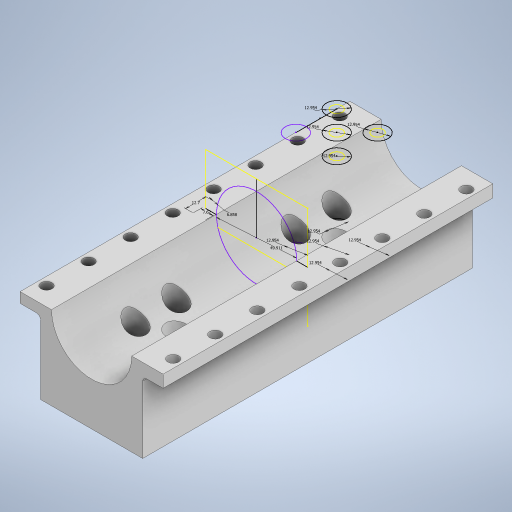
# Autodesk Inventor part: CameraHolder_LengthofTranslationStage
Saved by Autodesk Inventor 2024.2 (Build 282272000, 272)
## iProperties
Created: 2023-12-14
Part Number: CameraHolder_LengthofTranslationStage
Material: Generic
Document SubType Name: Modeling
Designer: S227943
Density: 1 g/cm^3
Appearance: Default
Author: S227943
Autodesk Inventor part; units mm, degrees
ref_plane "YZ Plane" through (0, 0, 0) normal (1, 0, 0) x (0, 1, 0)
ref_plane "XZ Plane" through (0, 0, 0) normal (0, 1, 0) x (-1, 0, 0)
ref_plane "XY Plane" through (0, 0, 0) normal (0, 0, 1) x (1, 0, 0)
sketch "Sketch1" plane through (0, 0, 0) normal (0, 1, 0) x (-1, 0, 0)
  line L0 (0, 0) -> (0, -102.499)
  line L1 (0, -102.499) -> (63.5, -102.499)
  line L2 (63.5, -102.499) -> (63.5, 0)
  line L3 (63.5, 0) -> (0, 0)
  dimension "d0" = 102.499
  dimension "d1" = 63.5
  constraints: 8 end point, 3 perpendicular, 1 vertical
  measures "d0" distance of L0.start L0.end
  measures "d1" distance of L0.end L1.end
extrude "Extrusion1" add sketch "Sketch1" along normal blind 63.5
sketch "Sketch2" plane through (-63.5, 0, 0) normal (0, 0, 1) x (1, 0, 0)
  line L0 (63.5, 63.5) -> (0, 63.5) projected
  line L1 (31.75, 63.5) -> (31.75, 31.75)
  circle A0 centre (31.75, 31.75) radius 24.9555
  line L2 (0, 0) -> (0, 63.5) projected
  line L3 (0, 31.75) -> (6.7945, 31.75)
  line L4 (63.5, 0) -> (63.5, 63.5) projected
  line L5 (63.5, 31.75) -> (56.7055, 31.75)
  dimension "d4" = 49.911
  constraints: 6 end point, 3 midpoint, 2 point on circle, 1 centre point, 1 coincident, 1 perpendicular, 1 point on line, 1 vertical
  measures "d4" diameter of A0
extrude "Extrusion2" cut sketch "Sketch2" against normal blind 139.7 contours A0
sketch "Sketch3" plane through (0, 0, 0) normal (1, 0, 0) x (0, 0, -1)
  line L0 (0, 0) -> (0, 63.5) projected
  line L1 (0, 31.75) -> (102.499, 31.75)
  line L2 (102.499, 0) -> (102.499, 63.5) projected
  constraints: 2 end point, 2 midpoint
split_face "Split1"
extrude "Extrusion3" cut sketch "Sketch2" against normal blind 139.7 contours L4 L5 A0 L1 L0 | L1 A0 L3 L2 L0
sketch "Sketch5" plane through (0, 0, 0) normal (0, -1, 0) x (1, 0, 0)
  line L0 (0, 0) -> (-31.75, 0)
  line L1 (-56.7055, 0) -> (-6.7945, 0) projected
  line L2 (-31.75, 0) -> (-31.75, -49.794)
  line L3 (0, 0) -> (0, -102.499) projected
  line L4 (-31.75, -49.794) -> (-19.05, -49.794)
  line L5 (-19.05, -49.794) -> (-19.05, -62.494)
  line L6 (-19.05, -62.494) -> (-44.45, -62.494)
  line L7 (-44.45, -62.494) -> (-44.45, -37.094)
  line L8 (-44.45, -37.094) -> (-19.05, -37.094)
  circle A0 centre (-19.05, -62.494) radius 3.429
  circle A1 centre (-44.45, -62.494) radius 3.429
  circle A2 centre (-19.05, -37.094) radius 3.429
  circle A3 centre (-44.45, -37.094) radius 3.429
  circle A4 centre (-31.75, -49.794) radius 3.429
  line L9 (-19.05, -62.494) -> (-19.05, -102.499)
  line L10 (0, -102.499) -> (-63.5, -102.499) projected
  dimension "d9" = 12.7
  dimension "d10" = 12.7
  dimension "d11" = 25.4
  dimension "d12" = 25.4
  dimension "d13" = 6.858
  dimension "d14" = 6.858
  dimension "d15" = 6.858
  dimension "d16" = 6.858
  dimension "d17" = 6.858
  dimension "d74" = 40.005
  constraints: 16 end point, 5 centre point, 5 coincident, 4 perpendicular, 2 point on line, 1 midpoint, 1 parallel, 1 vertical
  measures "d9" distance of L2.end L4.end
  measures "d10" distance of L4.end L5.end
  measures "d11" distance of L5.end L6.end
  measures "d12" distance of L6.end L7.end
  measures "d13" diameter of A0
  measures "d14" diameter of A1
  measures "d15" diameter of A2
  measures "d16" diameter of A3
  measures "d17" diameter of A4
  measures "d74" distance of L9.start L9.end
extrude "Extrusion4" cut sketch "Sketch5" against normal blind 139.7 contours L9 L5 A0 | A0 L6 L9 | A4 L4 L2 | L2 L4 A4 | A3 L7 L8 | L8 L7 A3 | A0 L5 L6 | A1 L7 L6 | L6 L7 A1 | A2
sketch "Sketch6" plane through (0, 0, 0) normal (0, -1, 0) x (1, 0, 0)
  circle A0 centre (-19.05, -37.094) radius 3.429 projected
  circle A1 centre (-44.45, -37.094) radius 3.429 projected
  line L0 (-19.05, -37.094) -> (-44.45, -37.094)
  circle A2 centre (-44.45, -62.494) radius 3.429 projected
  line L1 (-44.45, -37.094) -> (-44.45, -62.494)
  line L2 (-44.45, -62.494) -> (-19.05, -62.494)
  line L3 (-19.05, -62.494) -> (-31.75, -49.794)
  circle A3 centre (-19.05, -37.094) radius 6.477
  circle A4 centre (-31.75, -49.794) radius 6.477
  circle A5 centre (-44.45, -62.494) radius 6.477
  circle A6 centre (-19.05, -62.494) radius 6.477
  circle A7 centre (-44.45, -37.094) radius 6.477
  point P0 (0, 0)
  dimension "d20" = 12.954
  dimension "d21" = 12.954
  dimension "d22" = 12.954
  dimension "d23" = 12.954
  dimension "d24" = 12.954
  constraints: 8 end point, 5 centre point, 4 coincident, 2 perpendicular, 1 horizontal, 1 point on line
  measures "d20" diameter of A3
  measures "d21" diameter of A4
  measures "d22" diameter of A5
  measures "d23" diameter of A6
  measures "d24" diameter of A7
sketch "Sketch7" plane through (0, 63.5, 0) normal (0, 1, 0) x (1, 0, 0)
  circle A0 centre (-19.05, 37.094) radius 3.429 projected
  circle A1 centre (-19.05, 37.094) radius 6.477
  circle A2 centre (-31.75, 49.794) radius 3.429 projected
  circle A3 centre (-31.75, 49.794) radius 6.477
  circle A4 centre (-44.45, 62.494) radius 3.429 projected
  circle A5 centre (-44.45, 62.494) radius 6.477
  circle A6 centre (-19.05, 62.494) radius 3.429 projected
  circle A7 centre (-19.05, 62.494) radius 6.477
  line L0 (-44.45, 62.494) -> (-44.45, 52.2986)
  line L1 (-44.45, 62.494) -> (-44.45, 37.094)
  circle A8 centre (-44.45, 37.094) radius 6.477
  point P0 (0, 0)
  dimension "d25" = 12.954
  dimension "d26" = 12.954
  dimension "d28" = 12.954
  dimension "d29" = 12.954
  constraints: 5 centre point, 5 coincident, 4 end point, 2 vertical
  measures "d25" diameter of A1
  measures "d26" diameter of A3
  measures "d28" diameter of A5
  measures "d29" diameter of A7
extrude "Extrusion5" cut sketch "Sketch7" against normal blind 62.23 contours A0 | A1 | A2 | A3 | A4 | A5 | A6 | A7 | A8
sketch "Sketch8" plane through (-63.5, 0, -102.499) normal (-1, 0, 0) x (0, 0, 1)
  line L0 (102.499, 31.75) -> (0, 31.75) projected
  line L1 (0, 31.75) -> (0, 25.4)
  line L2 (0, 6.7945) -> (0, 31.75) projected
  line L3 (0, 25.4) -> (102.499, 25.4)
  line L4 (102.499, 25.4) -> (102.499, 31.75)
  line L5 (102.499, 31.75) -> (0, 31.75)
  point P0 (102.499, 0)
  dimension "d32" = 6.35
  dimension "d76" = 102.499
  constraints: 8 end point, 3 perpendicular, 1 point on line
  measures "d32" distance of L0.end L1.end
  measures "d76" distance of L1.end L3.end
extrude "Extrusion6" add sketch "Sketch8" along normal blind 12.7
sketch "Sketch9" plane through (-63.5, 25.4, -102.499) normal (0, -1, 0) x (1, 0, 0)
  line L0 (0, 102.499) -> (63.5, 102.499) projected
  line L1 (0, 102.499) -> (-7.62, 102.499)
  line L2 (-12.7, 102.499) -> (-12.7, 0) projected
  line L3 (-7.62, 102.499) -> (-7.62, 89.799)
  circle A0 centre (-7.62, 89.799) radius 3.429
  point P0 (-12.7, 129.9972)
  dimension "d35" = 7.62
  dimension "d36" = 12.7
  dimension "d37" = 6.858
  constraints: 4 end point, 2 perpendicular, 1 centre point, 1 coincident
  measures "d35" distance of L0.start L1.end
  measures "d36" distance of L1.end L3.end
  measures "d37" diameter of A0
extrude "Extrusion7" cut sketch "Sketch9" against normal blind 7.62
pattern_linear "Rectangular Pattern1" count 5 spacing -26.1493 along (0, 0, 1) of "Extrusion7"
sketch "Sketch10" plane through (0, 0, 0) normal (1, 0, 0) x (0, 0, -1)
  line L0 (102.499, 31.75) -> (102.499, 24.13)
  line L1 (102.499, 0) -> (102.499, 31.75) projected
  line L2 (102.499, 24.13) -> (0, 24.13)
  line L3 (0, 24.13) -> (0, 31.75)
  line L4 (0, 31.75) -> (102.499, 31.75)
  point P0 (0, 0)
  dimension "d43" = 7.62
  dimension "d75" = 102.499
  constraints: 8 end point, 3 perpendicular, 1 point on line
  measures "d43" distance of L0.start L0.end
  measures "d75" distance of L3.end L0.start
extrude "Extrusion8" add sketch "Sketch10" along normal blind 12.7
sketch "Sketch11" plane through (0, 24.13, -102.499) normal (0, -1, 0) x (1, 0, 0)
  line L0 (0, 102.499) -> (7.62, 102.499)
  line L1 (0, 102.499) -> (12.7, 102.499) projected
  line L2 (7.62, 102.499) -> (7.62, 89.799)
  circle A0 centre (7.62, 89.799) radius 3.429
  dimension "d46" = 7.62
  dimension "d47" = 12.7
  dimension "d48" = 6.858
  constraints: 4 end point, 1 centre point, 1 coincident, 1 perpendicular, 1 point on line
  measures "d46" distance of L0.start L0.end
  measures "d47" distance of L0.end L2.end
  measures "d48" diameter of A0
extrude "Extrusion9" cut sketch "Sketch11" against normal blind 12.7
pattern_linear "Rectangular Pattern2" count 5 spacing 26.1493 along (0, 0, -1) of "Extrusion9"
fillet "Fillet1" radius 2.54 2 edges at (0, 24.13, -51.2495) (-63.5, 25.4, -51.2495)
thicken "Thicken1" operation add thickness 20 both sides no extend neighbours no toward (0, -1, 0) faces at (-35.578, 0, -90.2327)
extrude "Extrusion10" cut sketch "Sketch7" against normal blind 76.2 contours A0 | A1 | A2 | A3 | A4 | A5 | A6 | A7 | A8
mirror "Mirror2" about plane through (-63.5, 0, 0) normal (0, 0, 1)
body "Solid1"
